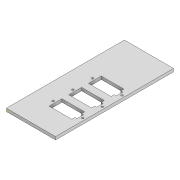
# Autodesk Inventor part: Part1_FInal
Saved by Autodesk Inventor 2020.2 (Build 242310000, 310)
## iProperties
Created: 2020-03-10
Part Number: Part1_FInal
Material: Generic
Document SubType Name: Modeling
Designer: Yash
Density: 1 g/cm^3
Appearance: Default
Author: Yash
Autodesk Inventor part; units mm, degrees
ref_plane "YZ Plane" through (0, 0, 0) normal (1, 0, 0) x (0, 1, 0)
ref_plane "XZ Plane" through (0, 0, 0) normal (0, 1, 0) x (-1, 0, 0)
ref_plane "XY Plane" through (0, 0, 0) normal (0, 0, 1) x (1, 0, 0)
sketch "Sketch1" plane through (0, 0, 0) normal (0, 1, 0) x (-1, 0, 0)
  point P0 (0, 0)
sketch "Sketch2" plane through (0, 0, 0) normal (0, 1, 0) x (-1, 0, 0)
  line L0 (0, 0) -> (-50, 0)
  line L1 (-50, 0) -> (-50, -120)
  line L2 (-50, -120) -> (0, -120)
  line L3 (0, -120) -> (0, 0)
  line L4 (-20, -23.5) -> (-43, -23.5)
  line L5 (-43, -23.5) -> (-43, -26.75)
  line L6 (-43, -26.75) -> (-45, -26.75)
  line L7 (-45, -26.75) -> (-45, -33.25)
  line L8 (-45, -33.25) -> (-43, -33.25)
  line L9 (-43, -33.25) -> (-43, -36.5)
  line L10 (-43, -36.5) -> (-20, -36.5)
  line L11 (-20, -36.5) -> (-20, -23.5)
  line L12 (-20, -43.5) -> (-43, -43.5)
  line L13 (-43, -43.5) -> (-43, -46.75)
  line L14 (-43, -46.75) -> (-45, -46.75)
  line L15 (-45, -46.75) -> (-45, -53.25)
  line L16 (-45, -53.25) -> (-43, -53.25)
  line L17 (-43, -53.25) -> (-43, -56.5)
  line L18 (-43, -56.5) -> (-20, -56.5)
  line L19 (-20, -56.5) -> (-20, -43.5)
  line L20 (-20, -63.5) -> (-43, -63.5)
  line L21 (-43, -63.5) -> (-43, -66.75)
  line L22 (-43, -66.75) -> (-45, -66.75)
  line L23 (-45, -66.75) -> (-45, -73.25)
  line L24 (-45, -73.25) -> (-43, -73.25)
  line L25 (-43, -73.25) -> (-43, -76.5)
  line L26 (-43, -76.5) -> (-20, -76.5)
  line L27 (-20, -76.5) -> (-20, -63.5)
  circle A0 centre (-17.5, -50) radius 1
  circle A1 centre (-17.5, -70) radius 1
  circle A2 centre (-17.5, -30) radius 1
  circle A3 centre (-47.4974, -30) radius 1
  circle A4 centre (-47.5, -50) radius 1
  circle A5 centre (-47.5, -70) radius 1
  dimension "d0" = 50
  dimension "d1" = 120
  dimension "d4" = 23
  dimension "d5" = 3.25
  dimension "d6" = 2
  dimension "d7" = 6.5
  dimension "d8" = 2
  dimension "d9" = 3.25
  dimension "d10" = 23
  dimension "d12" = 23
  dimension "d13" = 3.25
  dimension "d14" = 2
  dimension "d15" = 6.5
  dimension "d16" = 2
  dimension "d17" = 3.25
  dimension "d18" = 23
  dimension "d20" = 23
  dimension "d21" = 3.25
  dimension "d22" = 2
  dimension "d23" = 6.5
  dimension "d24" = 3.25
  dimension "d25" = 23
  dimension "d29" = 2
  dimension "d30" = 2
  dimension "d31" = 2
  dimension "d32" = 2
  dimension "d35" = 2
  dimension "d36" = 2
  constraints: 56 end point, 13 perpendicular, 6 centre point, 5 point on line, 2 horizontal, 2 parallel, 1 vertical
  measures "d0" distance of L2.end L1.end
  measures "d1" distance of L1.end L0.end
  measures "d4" distance of L4.start L4.end
  measures "d5" distance of L4.end L5.end
  measures "d6" distance of L5.end L6.end
  measures "d7" distance of L6.end L7.end
  measures "d8" distance of L7.end L8.end
  measures "d9" distance of L8.end L9.end
  measures "d10" distance of L9.end L10.end
  measures "d12" distance of L12.start L12.end
  measures "d13" distance of L12.end L13.end
  measures "d14" distance of L13.end L14.end
  measures "d15" distance of L14.end L15.end
  measures "d16" distance of L15.end L16.end
  measures "d17" distance of L16.end L17.end
  measures "d18" distance of L17.end L18.end
  measures "d20" distance of L20.start L20.end
  measures "d21" distance of L20.end L21.end
  measures "d22" distance of L21.end L22.end
  measures "d23" distance of L22.end L23.end
  measures "d24" distance of L24.end L25.end
  measures "d25" distance of L25.end L26.end
  measures "d29" diameter of A0
  measures "d30" diameter of A1
  measures "d31" diameter of A2
  measures "d32" diameter of A3
  measures "d35" diameter of A4
  measures "d36" diameter of A5
extrude "Extrusion1" add sketch "Sketch2" along normal blind 3
body "Solid1"
